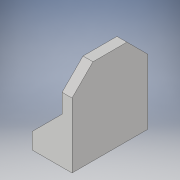
# Autodesk Inventor part: МД.001.1005 - Прихват
Saved by Autodesk Inventor 2019 (Build 230136000, 136)
## iProperties
Created: 2020-01-02
Part Number: МД.001.1005 - Прихват
Material: Типовые
Document SubType Name: Modeling
Designer: Петров Иван
Density: 1 g/cm^3
Appearance: По умолчанию
Author: Петров Иван
Autodesk Inventor part; units mm, degrees
ref_plane "YZ Plane" through (0, 0, 0) normal (1, 0, 0) x (0, 1, 0)
ref_plane "XZ Plane" through (0, 0, 0) normal (0, 1, 0) x (-1, 0, 0)
ref_plane "XY Plane" through (0, 0, 0) normal (0, 0, 1) x (1, 0, 0)
sketch "Эскиз1" plane through (0, 0, 0) normal (0, 1, 0) x (-1, 0, 0)
  line L0 (-10, 19) -> (10, 19)
  line L1 (10, 19) -> (10, -19)
  line L2 (10, -19) -> (-10, -19)
  line L3 (-10, -19) -> (-10, 19)
  line L4 (-10, 19) -> (10, -19) construction
  line L5 (10, 19) -> (-10, -19) construction
  circle A0 centre (0, 0) radius 5
  line L6 (0, 0) -> (0, 10)
  line L7 (0, 10) -> (0, -10)
  circle A1 centre (0, 10) radius 2
  circle A2 centre (0, -10) radius 2
  dimension "d0" = 20
  dimension "d1" = 38
  dimension "d2" = 10
  dimension "d3" = 10
  dimension "d4" = 20
  dimension "d5" = 4
  dimension "d6" = 4
  constraints: 16 end point, 3 centre point, 3 coincident, 2 midpoint, 2 parallel, 1 horizontal, 1 perpendicular, 1 point on line, 1 vertical
  measures "d0" distance of L1.end L2.end
  measures "d1" distance of L0.end L1.end
  measures "d2" diameter of A0
  measures "d3" distance of L6.start L6.end
  measures "d4" distance of L6.end L7.end
  measures "d5" diameter of A1
  measures "d6" diameter of A2
extrude "Выдавливание1" add sketch "Эскиз1" along normal blind 3
sketch "Эскиз2" plane through (0, 3, 0) normal (0, 1, 0) x (1, 0, 0)
  line L0 (-10, -19) -> (10, -19) projected
  line L1 (10, -19) -> (5, -19)
  line L2 (5, -19) -> (5, 19)
  line L3 (5, 19) -> (10, 19)
  line L4 (10, 19) -> (10, -19)
  point P0 (0, 0)
  dimension "d9" = 38
  dimension "d10" = 5
  constraints: 8 end point, 2 parallel, 1 horizontal, 1 perpendicular
  measures "d9" distance of L1.end L2.end
  measures "d10" distance of L2.end L3.end
extrude "Выдавливание2" add sketch "Эскиз2" along normal blind 40
chamfer "Фаска1" distance 10.5 angle 45 2 edges at (7.5, 43, -19) (7.5, 43, 19)
sketch "Эскиз3" plane through (0, 3, 0) normal (0, 1, 0) x (1, 0, 0)
  line L0 (-10, 19) -> (10, 19) projected
  line L1 (5, 0) -> (5, 19) projected
  line L2 (-10, 19) -> (5, 19)
  line L3 (5, 19) -> (5, 14)
  line L4 (5, 14) -> (-10, 14)
  line L5 (-10, 14) -> (-10, 19)
  line L6 (10, -19) -> (-10, -19) projected
  line L7 (5, -8.5) -> (5, -19) projected
  line L8 (-10, -19) -> (5, -19)
  line L9 (5, -19) -> (5, -14)
  line L10 (5, -14) -> (-10, -14)
  line L11 (-10, -14) -> (-10, -19)
  point P0 (0, 0)
  dimension "d16" = 5
  dimension "d17" = 5
  constraints: 16 end point, 4 parallel, 2 horizontal, 2 perpendicular, 2 point on line
  measures "d16" distance of L2.end L3.end
  measures "d17" distance of L9.end L8.end
extrude "Выдавливание3" add sketch "Эскиз3" along normal blind 20
chamfer "Фаска2" distance 15 angle 45 2 edges at (-10, 23, -16.5) (-10, 23, 16.5)
